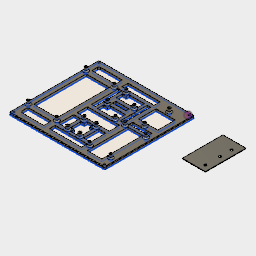
Thrower Case (Autodesk Fusion 360 design; units mm, degrees)
Autodesk Fusion 360 part; units mm, degrees
sketch "Sketch1" plane through (0, 0, 0) normal (0, 1, 0) x (1, 0, 0)
  line L0 (10, -2.6) -> (10, -148.4)
  circle A0 centre (5, -2.5) radius 1.55
  circle A1 centre (5, -148.5) radius 1.55
  line L1 (-153, -145.5014) -> (-153, -150.5334)
  line L2 (-150.4, -153.1334) -> (7.4, -153.1334)
  line L3 (10, -150.5334) -> (10, -142.9732)
  circle A2 centre (-150.5, -148.5) radius 1.55
  arc A3 (7.4, -153.1334) -> (10, -150.5334) centre (7.4, -150.5334) ccw
  line L4 (-155, -8) -> (-155, -0.6)
  line L5 (-152.4, 2) -> (7.4, 2)
  line L6 (10, -0.6) -> (10, -8)
  circle A4 centre (-150.5, -2.5) radius 1.55
  line L7 (-150.4, 2) -> (-145, 2)
  line L8 (-143, -153.1334) -> (-152.4, -153.1334)
  line L9 (-155, -150.5334) -> (-155, -0.6)
  arc A5 (10, -0.6) -> (7.4, 2) centre (7.4, -0.6) ccw
  arc A6 (-142.4, -8) -> (-145, -10.6) centre (-142.4, -10.6) ccw
  arc A7 (-155, -150.5334) -> (-152.4, -153.1334) centre (-152.4, -150.5334) ccw
  arc A8 (-145, -140.3014) -> (-142.4, -142.9014) centre (-142.4, -140.3014) ccw
  arc A9 (-152.4, 2) -> (-155, -0.6) centre (-152.4, -0.6) ccw
  line L10 (-145, -20) -> (-105, -20)
  line L11 (-105, -130) -> (-145, -130)
  line L12 (-155, -130) -> (-155, -20)
  line L13 (-145, -30) -> (-105, -30)
  line L14 (-105, -30) -> (-105, -120)
  line L15 (-105, -120) -> (-145, -120)
  line L16 (-145, -120) -> (-145, -30)
  line L17 (-145, -10.6) -> (-145, -20)
  line L18 (-145, -30) -> (-145, -120)
  line L19 (-145, -130) -> (-145, -140.3014)
  circle A10 centre (-150, -25.5) radius 2.5
  circle A11 centre (-101, -25.5) radius 2.5
  circle A12 centre (-150, -124.5) radius 2.5
  circle A13 centre (-101, -124.5) radius 2.5
  circle A14 centre (-150, -25.5) radius 1.4
  circle A15 centre (-101, -25.5) radius 1.4
  circle A16 centre (-101, -124.5) radius 1.4
  circle A17 centre (-150, -124.5) radius 1.4
  line L20 (-30, -73) -> (-5, -73)
  line L21 (-5, -73) -> (-5, -143)
  line L22 (-5, -143) -> (-30, -143)
  line L23 (-30, -143) -> (-30, -73)
  circle A18 centre (-35, -73) radius 2.5
  circle A19 centre (1, -73) radius 2.5
  circle A20 centre (-35.2709, -133.5) radius 2.5
  circle A21 centre (0.7291, -133.5) radius 2.5
  circle A22 centre (-35, -73) radius 1.4
  circle A23 centre (1, -73) radius 1.4
  circle A24 centre (0.7291, -133.5) radius 1.4
  circle A25 centre (-35.2709, -133.5) radius 1.4
  line L24 (-40, -138) -> (-40, -142.9014)
  line L25 (-105, -130) -> (-105, -142.9014)
  line L26 (-95, -142.9014) -> (-95, -133.2772)
  line L27 (-105, -20) -> (-105, -8)
  line L28 (-95, -8) -> (-95, -18.2401)
  line L29 (-105, -8) -> (-142.4, -8)
  line L30 (-40, -142.9014) -> (-95, -142.9014)
  line L31 (-105, -142.9014) -> (-142.4, -142.9014)
  circle A26 centre (-17, -15) radius 2.5
  circle A27 centre (-17, -57.5) radius 2.5
  line L32 (0, -52) -> (0, -22)
  line L33 (-33, -22) -> (0, -22)
  line L34 (0, -22) -> (0, -52)
  line L35 (0, -52) -> (-33, -52)
  line L36 (-33, -52) -> (-33, -22)
  line L37 (-33, -62) -> (0, -62)
  line L38 (0, -62) -> (0, -68)
  line L39 (0, -68) -> (-33, -68)
  line L40 (-33, -68) -> (-33, -62)
  circle A28 centre (-17, -15) radius 1.4
  circle A29 centre (-17, -57.5) radius 1.4
  circle A30 centre (-52.3216, -39.9901) radius 2.5
  line L41 (-55.8216, -45.2401) -> (-78.8216, -45.2401)
  line L42 (-88.8216, -45.2401) -> (-88.8216, -24.2401)
  line L43 (-76.8216, -29.1946) -> (-76.8216, -24.2401)
  line L44 (-58.8216, -34.2401) -> (-50.8216, -34.2401)
  circle A31 centre (-82.3216, -23.4901) radius 1.4
  line L45 (-45.8216, -24.2401) -> (-45.8216, -45.2401)
  line L46 (-50.8216, -34.2401) -> (-50.8216, -24.2401)
  line L47 (-76.8216, -29.1946) -> (-83.8216, -29.1946)
  line L48 (-83.8216, -29.1946) -> (-83.8216, -39.2401)
  line L49 (-58.8216, -39.2401) -> (-76.8216, -39.2401)
  line L50 (-83.8216, -39.2401) -> (-76.8216, -39.2401)
  circle A32 centre (-52.3216, -39.9901) radius 1.4
  line L51 (-76.8216, -24.2401) -> (-58.8216, -24.2401)
  circle A33 centre (-82.3216, -23.4901) radius 2.5
  line L52 (-78.8216, -18.2401) -> (-55.8216, -18.2401)
  line L53 (-58.8216, -34.2401) -> (-58.8216, -39.2401)
  line L54 (-50.8216, -24.2401) -> (-58.8216, -24.2401)
  circle A34 centre (-52.3382, -72.4785) radius 2.5
  line L55 (-45.8382, -77.7285) -> (-88.8382, -77.7285)
  line L56 (-88.8382, -70.7285) -> (-88.8382, -50.7285)
  line L57 (-76.8382, -61.683) -> (-76.8382, -56.7285)
  line L58 (-58.8382, -66.7285) -> (-50.8382, -66.7285)
  circle A35 centre (-82.3382, -55.9785) radius 1.4
  line L59 (-45.8382, -50.7285) -> (-45.8382, -70.7285)
  line L60 (-50.8382, -66.7285) -> (-50.8382, -56.7285)
  line L61 (-76.8382, -61.683) -> (-83.8382, -61.683)
  line L62 (-83.8382, -61.683) -> (-83.8382, -71.7285)
  line L63 (-58.8382, -71.7285) -> (-76.8382, -71.7285)
  line L64 (-83.8382, -71.7285) -> (-76.8382, -71.7285)
  circle A36 centre (-52.3382, -72.4785) radius 1.4
  line L65 (-76.8382, -56.7285) -> (-58.8382, -56.7285)
  circle A37 centre (-82.3382, -55.9785) radius 2.5
  line L66 (-58.8382, -66.7285) -> (-58.8382, -71.7285)
  line L67 (-50.8382, -56.7285) -> (-58.8382, -56.7285)
  line L68 (-40, -8) -> (-45.8216, -8)
  line L69 (-55.8216, -8) -> (-78.8216, -8)
  line L70 (-88.8216, -8) -> (-95, -8)
  line L71 (-78.8216, -45.2401) -> (-78.8216, -50.7285)
  line L72 (-88.8216, -50.7285) -> (-88.8216, -45.2401)
  line L73 (-55.8216, -45.2401) -> (-55.8216, -50.7285)
  line L74 (-45.8382, -50.7285) -> (-45.8216, -50.7285)
  line L75 (-45.8216, -50.7285) -> (-45.8216, -45.2401)
  line L76 (-88.8382, -50.7285) -> (-88.8216, -50.7285)
  line L77 (-78.8216, -50.7285) -> (-55.8216, -50.7285)
  line L78 (-88.8382, -77.7285) -> (-95, -77.7285)
  line L79 (-95, -70.7285) -> (-88.8382, -70.7285)
  line L80 (-45.8382, -77.7285) -> (-40, -77.7285)
  line L81 (-40, -70.7285) -> (-45.8382, -70.7285)
  line L82 (-95, -24.2401) -> (-95, -70.7285)
  line L83 (-40, -69.5) -> (-40, -70.7285)
  line L84 (-55.8216, -18.2401) -> (-45.8216, -18.2401)
  line L85 (-50.8216, -24.2401) -> (-55.8216, -24.2401)
  line L86 (-88.8216, -18.2401) -> (-95, -18.2401)
  line L87 (-95, -24.2401) -> (-88.8216, -24.2401)
  line L88 (-88.8216, -8) -> (-78.8216, -8)
  line L89 (-55.8216, -8) -> (-45.8216, -8)
  line L90 (-78.8216, -18.2401) -> (-88.8216, -18.2401)
  line L91 (-45.8216, -18.2401) -> (-40, -18.2401)
  line L92 (-40, -24.2401) -> (-45.8216, -24.2401)
  line L93 (-40, -8) -> (-40, -18.2401)
  line L94 (-40, -24.2401) -> (-40, -69.5)
  circle A38 centre (-57.4742, -100.2772) radius 1.45
  line L95 (-78.4742, -122.7772) -> (-78.4742, -105.7772)
  circle A39 centre (-78.4742, -100.2772) radius 3
  circle A40 centre (-57.4742, -100.2772) radius 3
  line L96 (-78.4742, -105.7772) -> (-72.4742, -105.7772)
  line L97 (-63.4742, -105.7772) -> (-57.4742, -105.7772)
  line L98 (-72.4742, -99.7772) -> (-63.4742, -99.7772)
  line L99 (-57.4742, -105.7772) -> (-57.4742, -122.7772)
  circle A41 centre (-78.4742, -100.2772) radius 1.45
  line L100 (-72.4742, -105.7772) -> (-72.4742, -99.7772)
  line L101 (-63.4742, -99.7772) -> (-63.4742, -105.7772)
  line L102 (-72.4742, -122.7772) -> (-78.4742, -122.7772)
  circle A42 centre (-78.4742, -128.2772) radius 1.45
  circle A43 centre (-78.4742, -128.2772) radius 3
  line L103 (-57.4742, -122.7772) -> (-63.4742, -122.7772)
  line L104 (-63.4742, -128.7772) -> (-72.4742, -128.7772)
  line L105 (-72.4742, -128.7772) -> (-72.4742, -122.7772)
  line L106 (-63.4742, -122.7772) -> (-63.4742, -128.7772)
  circle A44 centre (-57.4742, -128.2772) radius 1.45
  line L107 (-83.9742, -95.2772) -> (-51.9742, -95.2772)
  circle A45 centre (-57.4742, -128.2772) radius 3
  line L108 (-51.9742, -101.2772) -> (-51.9742, -127.2772)
  line L109 (-51.9742, -133.2772) -> (-83.9742, -133.2772)
  line L110 (-83.9742, -127.2772) -> (-83.9742, -101.2772)
  line L111 (-83.9742, -133.2772) -> (-95, -133.2772)
  line L112 (-95, -127.2772) -> (-83.9742, -127.2772)
  line L113 (-51.9742, -133.2772) -> (-40, -133.2772)
  line L114 (-40, -127.2772) -> (-51.9742, -127.2772)
  line L115 (-51.9742, -95.2772) -> (-40, -95.2772)
  line L116 (-40, -101.2772) -> (-51.9742, -101.2772)
  line L117 (-83.9742, -95.2772) -> (-95, -95.2772)
  line L118 (-95, -101.2772) -> (-83.9742, -101.2772)
  line L119 (-40, -77.7285) -> (-40, -95.2772)
  line L120 (-40, -101.2772) -> (-40, -127.2772)
  line L121 (-40, -133.2772) -> (-40, -138)
  line L122 (-95, -77.7285) -> (-95, -95.2772)
  line L123 (-95, -101.2772) -> (-95, -127.2772)
  point P0 (10, 0)
  point P1 (0, -151)
  point P2 (-153, -142.9014)
  point P3 (-155, 2)
  point P4 (10, 2)
  dimension "d1" = 10
  dimension "d5" = 3.1
  dimension "d7" = 3.1
  dimension "d11" = 5
  dimension "d12" = 5
  dimension "d19" = 3.1
  dimension "d20" = 2.5
  dimension "d23" = 2.6
  dimension "d27" = 4.6334
  dimension "d28" = 4.6334
  dimension "d30" = 10
  dimension "d32" = 4.5
  dimension "d33" = 3.1
  dimension "d34" = 4.5
  dimension "d35" = 4.5
  dimension "d36" = 10
  dimension "d37" = 155.1334
  dimension "d38" = 2.6
  dimension "d41" = 2.6
  dimension "d42" = 2.6
  dimension "d43" = 2.6
  dimension "d44" = 165
  dimension "d45" = 2.6
  dimension "d46" = 10
  dimension "d47" = 4.5
  dimension "d247" = 110
  dimension "d248" = 40
  dimension "d249" = 90
  dimension "d250" = 12
  dimension "d251" = 10
  dimension "d252" = 5
  dimension "d253" = 5
  dimension "d254" = 49
  dimension "d255" = 5
  dimension "d256" = 5
  dimension "d257" = 49
  dimension "d258" = 99
  dimension "d259" = 5.5
  dimension "d260" = 2.8
  dimension "d261" = 2.8
  dimension "d262" = 2.8
  dimension "d263" = 2.8
  dimension "d271" = 25
  dimension "d272" = 70
  dimension "d273" = 10
  dimension "d275" = 5
  dimension "d276" = 5
  dimension "d277" = 5
  dimension "d278" = 5
  dimension "d279" = 36
  dimension "d280" = 36
  dimension "d281" = 60.5
  dimension "d284" = 2.8
  dimension "d285" = 2.8
  dimension "d286" = 2.8
  dimension "d287" = 2.8
  dimension "d293" = 5
  dimension "d294" = 5
  dimension "d295" = 42.5
  dimension "d296" = 7
  dimension "d300" = 27
  dimension "d301" = 27
  dimension "d302" = 2.8
  dimension "d303" = 2.8
  dimension "d307" = 5
  dimension "d308" = 5
  dimension "d309" = 43
  dimension "d310" = 27
  dimension "d311" = 5.25
  dimension "d312" = 6.5
  dimension "d313" = 6.5
  dimension "d314" = 5.25
  dimension "d315" = 2.8
  dimension "d316" = 2.8
  dimension "d317" = 10
  dimension "d318" = 6
  dimension "d319" = 15
  dimension "d320" = 5
  dimension "d321" = 5
  dimension "d322" = 5
  dimension "d323" = 5
  dimension "d324" = 43
  dimension "d325" = 27
  dimension "d326" = 5.25
  dimension "d327" = 6.5
  dimension "d328" = 6.5
  dimension "d329" = 5.25
  dimension "d330" = 2.8
  dimension "d331" = 2.8
  dimension "d332" = 10
  dimension "d333" = 6
  dimension "d334" = 15
  dimension "d335" = 5
  dimension "d336" = 5
  dimension "d337" = 10
  dimension "d339" = 10
  dimension "d340" = 10
  dimension "d343" = 7
  dimension "d344" = 7
  dimension "d345" = 6
  dimension "d346" = 6
  dimension "d347" = 6
  dimension "d349" = 32
  dimension "d350" = 38
  dimension "d351" = 6
  dimension "d352" = 6
  dimension "d353" = 6
  dimension "d354" = 6
  dimension "d355" = 2.9
  dimension "d356" = 2.9
  dimension "d357" = 2.9
  dimension "d358" = 2.9
  dimension "d359" = 21
  dimension "d360" = 21
  dimension "d361" = 28
  dimension "d362" = 5.5
  dimension "d363" = 5
  dimension "d364" = 21
  dimension "d365" = 4.5
  dimension "d366" = 5.5
  dimension "d367" = 6
  dimension "d368" = 6
  dimension "d369" = 6
  dimension "d370" = 6
  measures "d1" distance of origin P0
  measures "d5" diameter of A0
  measures "d7" diameter of A1
  measures "d11" distance of L0 A1.centre
  measures "d12" distance of L0 A0.centre
  measures "d19" diameter of A2
  measures "d20" distance of L1 A2.centre
  measures "d23" radius of A3
  measures "d27" distance of A1.centre L2
  measures "d28" distance of L2 A2.centre
  measures "d30" distance of L6.end P4
  measures "d32" distance of A0.centre L5
  measures "d33" diameter of A4
  measures "d34" distance of L5 A4.centre
  measures "d35" distance of L4 A4.centre
  measures "d36" distance of P3 L7.end
  measures "d37" distance of L2 L5
  measures "d38" radius of A5
  measures "d41" radius of A6
  measures "d42" radius of A7
  measures "d43" radius of A8
  measures "d44" distance of L0 L9
  measures "d45" radius of A9
  measures "d46" distance of L9 L17
  measures "d47" distance of A2.centre L9
  measures "d247" distance of L12.end L12.start
  measures "d248" distance of L13.start L13.end
  measures "d249" distance of L13.start L15.end
  measures "d250" distance of L10 L68
  measures "d251" distance of L10 L13
  measures "d252" diameter of A10
  measures "d253" diameter of A11
  measures "d254" distance of A10.centre A11.centre
  measures "d255" diameter of A12
  measures "d256" diameter of A13
  measures "d257" distance of A12.centre A13.centre
  measures "d258" distance of A10.centre A12.centre
  measures "d259" distance of L10 A11.centre
  measures "d260" diameter of A14
  measures "d261" diameter of A15
  measures "d262" diameter of A16
  measures "d263" diameter of A17
  measures "d271" distance of L20.start L20.end
  measures "d272" distance of L20.start L22.end
  measures "d273" distance of L23 L83
  measures "d275" diameter of A18
  measures "d276" diameter of A19
  measures "d277" diameter of A20
  measures "d278" diameter of A21
  measures "d279" distance of A18.centre A19.centre
  measures "d280" distance of A20.centre A21.centre
  measures "d281" distance of A18.centre A20.centre
  measures "d284" diameter of A22
  measures "d285" diameter of A23
  measures "d286" diameter of A24
  measures "d287" diameter of A25
  measures "d293" diameter of A26
  measures "d294" diameter of A27
  measures "d295" distance of A26.centre A27.centre
  measures "d296" distance of A26.centre L68
  measures "d300" distance of L0 A27.centre
  measures "d301" distance of L0 A26.centre
  measures "d302" diameter of A28
  measures "d303" diameter of A29
  measures "d307" diameter of A33
  measures "d308" diameter of A30
  measures "d309" distance of L42.start L45.end
  measures "d310" distance of L42.start L86.start
  measures "d311" distance of A31.centre L52
  measures "d312" distance of A31.centre L42
  measures "d313" distance of A30.centre L45
  measures "d314" distance of A30.centre L41
  measures "d315" diameter of A31
  measures "d316" diameter of A32
  measures "d317" distance of L44 L54
  measures "d318" distance of L51 L52
  measures "d319" distance of L49 L51
  measures "d320" distance of L42 L48
  measures "d321" distance of L45 L46
  measures "d322" diameter of A37
  measures "d323" diameter of A34
  measures "d324" distance of L55.end L55.start
  measures "d325" distance of L55.end L56.end
  measures "d326" distance of A35.centre L76
  measures "d327" distance of A35.centre L56
  measures "d328" distance of A34.centre L59
  measures "d329" distance of A34.centre L55
  measures "d330" diameter of A35
  measures "d331" diameter of A36
  measures "d332" distance of L58 L67
  measures "d333" distance of L65 L76
  measures "d334" distance of L63 L65
  measures "d335" distance of L56 L62
  measures "d336" distance of L59 L60
  measures "d337" distance of L86.start L52.start
  measures "d339" distance of L42.start L41.end
  measures "d340" distance of L45.end L41.start
  measures "d343" distance of L55.end L56.start
  measures "d344" distance of L55.start L59.end
  measures "d345" distance of L52.end L85.end
  measures "d346" distance of L86.start L42.end
  measures "d347" distance of L84.end L45.start
  measures "d349" distance of L107.start L107.end
  measures "d350" distance of L107.start L109.end
  measures "d351" diameter of A39
  measures "d352" diameter of A40
  measures "d353" diameter of A43
  measures "d354" diameter of A45
  measures "d355" diameter of A41
  measures "d356" diameter of A38
  measures "d357" diameter of A44
  measures "d358" diameter of A42
  measures "d359" distance of A39.centre A38.centre
  measures "d360" distance of A42.centre A44.centre
  measures "d361" distance of A42.centre A39.centre
  measures "d362" distance of A39.centre L110
  measures "d363" distance of A39.centre L107
  measures "d364" distance of L95 L99
  measures "d365" distance of L98 L107
  measures "d366" distance of L99 L108
  measures "d367" distance of L109.end L110.start
  measures "d368" distance of L109.start L108.end
  measures "d369" distance of L107.end L108.start
  measures "d370" distance of L107.start L110.end
extrude "Extrude37" add sketch "Sketch1" along normal blind 10 contours A39 | A40 | A43 | A45 makes body 1 at (-77.6617, 6.6667, 97.3894) makes body 2 at (-75.8396, 3.3333, 126.8425) makes body 3 at (-54.8396, 3.3333, 98.8425) makes body 4 at (-60.3815, 6.6667, 127.537)
extrude "Extrude36" add sketch "Sketch1" along normal blind 10 separate body contours A30 | A33 | A34 | A37 makes body 5 at (-49.8989, 6.6667, 39.3732) makes body 6 at (-79.8413, 6.6667, 56.1031) makes body 7 at (-79.8247, 6.6667, 23.6147) makes body 8 at (-49.8413, 6.6667, 72.6031)
extrude "Extrude35" add sketch "Sketch1" along normal blind 10 separate body contours A26 | A27 makes body 9 at (-14.5031, 6.6667, 15.1246) makes body 10 at (-14.5031, 6.6667, 57.6246)
extrude "Extrude34" add sketch "Sketch1" along normal blind 10 separate body contours A18 | A19 | A20 | A21 makes body 11 at (3.1518, 6.6667, 134.1169) makes body 12 at (-1.3492, 6.6667, 73.8551) makes body 13 at (-32.8482, 6.6667, 132.8831) makes body 14 at (-37.3492, 6.6667, 73.8551)
extrude "Extrude32" add sketch "Sketch1" along normal blind 10 separate body contours A10 | A11 | A12 | A13 makes body 15 at (-150.7962, 6.6667, 122.1302) makes body 16 at (-149.3229, 6.6667, 23.0934) makes body 17 at (-103.4876, 6.6667, 124.7489) makes body 18 at (-98.5031, 6.6667, 25.6246)
extrude "Extrude33" add sketch "Sketch1" along normal blind 4 separate body contours L0 L2 L3 A3 L4 L5 L6 L7 L8 L9 A5 A7 A9 L12 | A18 | A19 | A20 | A21 | A22 | A23 | A24 | A25 | A26 | A27 | A28 | A29 | A30 | A31 | A32 | A33 | A34 | A35 | A36 | A37 | A38 | A39 | A40 | A41 | A42 | A43 | A44 | A45 makes body 19
combine "Combine7" operation add target body 17 tool bodies 19 15 18 16
fillet "Fillet13" radius 2 4 edges at (-152.3308, 4, 24.596) (-103.3308, 4, 24.596) (-103.3308, 4, 125.404) (-152.3308, 4, 123.596) on bodies 17
combine "Combine8" operation add target body 17 tool bodies 12 14 13 11
fillet "Fillet14" radius 2 4 edges at (-1.3308, 4, 72.096) (-1.6018, 4, 132.596) (-37.6018, 4, 132.596) (-37.3308, 4, 72.096) on bodies 17
combine "Combine9" operation add target body 17 tool bodies 10 9
fillet "Fillet15" radius 2 2 edges at (-19.3308, 4, 14.096) (-19.3308, 4, 56.596) on bodies 17
combine "Combine10" operation add target body 17 tool bodies 5 7 6 8
fillet "Fillet16" radius 2 4 edges at (-84.6524, 4, 22.5861) (-84.669, 4, 55.0745) (-54.6524, 4, 39.0861) (-54.669, 4, 71.5745) on bodies 17
combine "Combine11" operation add target body 17 tool bodies 1 2 3 4
fillet "Fillet17" radius 2 4 edges at (-60.2712, 4, 99.1924) (-81.2712, 4, 99.1924) (-81.2712, 4, 127.1924) (-60.2712, 4, 127.1924) on bodies 17
fillet "Fillet18" radius 1 9 edges at (-155, 4, 75.5667) (-154.2385, 4, 152.3718) (-147.7, 4, 153.1334) (-67.8, 4, 153.1334) (9.2385, 4, 152.3719) (10, 4, 75.5667) (9.2385, 4, -1.2385) (-72.5, 4, -2) (-154.2385, 4, -1.2385) on bodies 17
extrude "Extrude38" cut 14 faces at (-83.0175, 4, 55.6103) (-82.555, 4, 23.2594) (-51.8602, 4, 40.3255) (-53.0648, 4, 72.7414) (-35.0349, 4, 72.6571) (-17.5653, 4, 57.1146) (0.6939, 4, 72.5346) (-17.0349, 4, 14.5966) (-78.1729, 4, 99.4799) (-78.7159, 4, 128.9807) (-57.4381, 4, 127.2507) (-57.6508, 4, 99.4079) (-35.3058, 4, 134.6002) (0.6942, 4, 134.6002) along direction (0, 1, 0) mid plane 12 on bodies 17 bodies 17
sketch "Sketch7" plane through (0, 0, 0) normal (0, 1, 0) x (1, 0, 0)
  line L0 (60, 0) -> (100, 0)
  line L1 (100, 0) -> (100, -70)
  line L2 (100, -70) -> (60, -70)
  line L3 (60, -70) -> (60, 0)
  circle A0 centre (90, -15) radius 4
  circle A1 centre (90, -35) radius 4
  circle A2 centre (90, -60) radius 6
  circle A3 centre (90, -15) radius 2
  circle A4 centre (90, -35) radius 2
  circle A5 centre (90, -60) radius 2
  dimension "d377" = 40
  dimension "d378" = 70
  dimension "d379" = 8
  dimension "d380" = 8
  dimension "d381" = 12
  dimension "d382" = 15
  dimension "d383" = 30
  dimension "d384" = 30
  dimension "d385" = 30
  dimension "d386" = 20
  dimension "d387" = 25
  dimension "d388" = 4
  dimension "d389" = 4
  dimension "d390" = 4
  measures "d377" distance of L0.start L0.end
  measures "d378" distance of L0.start L2.end
  measures "d379" diameter of A0
  measures "d380" diameter of A1
  measures "d381" diameter of A2
  measures "d382" distance of L0 A0.centre
  measures "d383" distance of L3 A0.centre
  measures "d384" distance of L3 A1.centre
  measures "d385" distance of L3 A2.centre
  measures "d386" distance of A0.centre A1.centre
  measures "d387" distance of A1.centre A2.centre
  measures "d388" diameter of A3
  measures "d389" diameter of A4
  measures "d390" diameter of A5
extrude "Extrude39" add sketch "Sketch7" along normal blind 1 separate body contours L0 L1 L2 L3 | A0 | A1 | A2 makes body 20
